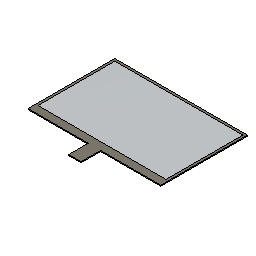
InfoWindow-Fusion360 (Autodesk Fusion 360 archive; units mm, degrees)
design "WS_Screen 7.5"
Autodesk Fusion 360 part; units mm, degrees
sketch "Sketch1" plane through (0, 0, 0) normal (0, 1, 0) x (1, 0, 0)
  line L0 (-84.9312, -55.5) -> (-84.9312, 55.5)
  line L1 (-84.9312, 55.5) -> (84.9312, 55.5)
  line L2 (84.9312, 55.5) -> (84.9312, -55.5)
  line L3 (84.9312, -55.5) -> (-84.9312, 55.5) construction
  line L4 (-84.9312, -55.5) -> (84.9312, 55.5) construction
  line L5 (0, 0) -> (0, -80) construction
  line L6 (-7.9312, -55.5) -> (-7.9312, -80.5)
  line L7 (7.9312, -55.5) -> (7.9312, -80.5)
  line L8 (-7.9312, -80.5) -> (7.9312, -80.5)
  line L9 (84.9312, -55.5) -> (7.9312, -55.5)
  line L10 (-7.9312, -55.5) -> (-84.9312, -55.5)
  dimension "d1" = 169.8625
  dimension "d2" = 111
  dimension "d3" = 77
  dimension "d4" = 77
  dimension "d5" = 25
  constraint perpendicular L0 L9
  constraint parallel L1 L9
  constraint parallel L0 L2
  constraint horizontal L9
  constraint coincident L3 L5.start
  constraint coincident L4 L5.start
  constraint coincident L5.start origin
  constraint perpendicular L5 L9
  constraint coincident L6.start L9
  constraint perpendicular L6 L9
  constraint perpendicular L7 L9
  constraint perpendicular L7 L8
  constraint collinear L9 L10
  measures "d1" distance of L0.end L1.end
  measures "d2" distance of L0.start L0.end
  measures "d3" distance of L2 L7
  measures "d4" distance of L0 L6 L2.end
  measures "d5" distance of L8 L9
extrude "Extrude1" add sketch "Sketch1" along normal blind 1.2
sketch "Sketch2" plane through (0, 1.2, 0) normal (0, 1, 0) x (-1, 0, 0)
  line L0 (7.9312, 80.5) -> (-7.9312, 80.5)
  line L1 (-7.9312, 80.5) -> (-7.9312, 55.5)
  line L2 (-7.9312, 55.5) -> (-84.9312, 55.5)
  line L3 (-84.9312, 55.5) -> (-84.9312, -55.5)
  line L4 (-84.9312, -55.5) -> (84.9312, -55.5)
  line L5 (84.9312, -55.5) -> (84.9312, 55.5)
  line L6 (84.9312, 55.5) -> (7.9312, 55.5)
  line L7 (7.9312, 55.5) -> (7.9312, 80.5)
  line L8 (-81.9312, 45.75) -> (81.9312, 45.75)
  line L9 (81.9312, 45.75) -> (81.9312, -52.5)
  line L10 (81.9312, -52.5) -> (-81.9312, -52.5)
  line L11 (-81.9312, -52.5) -> (-81.9312, 45.75)
  dimension "d8" = 3
  dimension "d9" = 3
  dimension "d10" = 3
  dimension "d11" = 9.75
  constraint perpendicular L8 L9
  constraint parallel L8 L10
  constraint parallel L9 L11
  constraint horizontal L8
  measures "d8" distance of L3 L11
  measures "d9" distance of L4 L10
  measures "d10" distance of L5 L9
  measures "d11" distance of L6 L8
extrude "Extrude2" add sketch "Sketch2" along normal blind 0.0001 contours L8 L9 L10 L11
equation "d1 = 6 11/16\""
